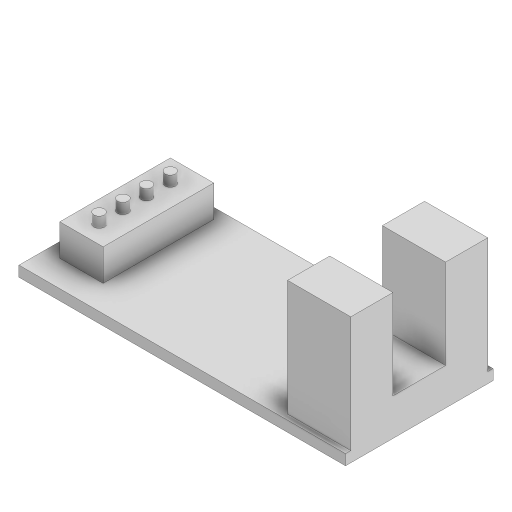
# Autodesk Inventor part: LM393
Saved by Autodesk Inventor 2024 (Build 280153000, 153)
## iProperties
Created: 2024-06-06
Part Number: LM393
Material: 一般
Document SubType Name: Modeling
Designer: USER
Density: 1 g/cm^3
Appearance: 預設
Author: USER
Autodesk Inventor part; units mm, degrees
ref_plane "YZ Plane" through (0, 0, 0) normal (1, 0, 0) x (0, 1, 0)
ref_plane "XZ Plane" through (0, 0, 0) normal (0, 1, 0) x (-1, 0, 0)
ref_plane "XY Plane" through (0, 0, 0) normal (0, 0, 1) x (1, 0, 0)
sketch "草圖1" plane through (0, 0, 0) normal (0, 1, 0) x (-1, 0, 0)
  line L0 (0, 0) -> (31, 0)
  line L1 (31, 0) -> (31, -14)
  line L2 (31, -14) -> (0, -14)
  line L3 (0, -14) -> (0, 0)
  line L4 (6, 0) -> (6, -14)
  line L5 (6, -0.5) -> (0, -0.5)
  line L6 (6, -4.5) -> (0, -4.5)
  line L7 (6, -13.5) -> (0, -13.5)
  line L8 (6, -9.5) -> (0, -9.5)
  line L9 (29.6283, -2.5) -> (25.5101, -2.5)
  line L10 (25.5101, -2.5) -> (25.5101, -13)
  line L11 (25.5101, -13) -> (29.6283, -13)
  line L12 (29.6283, -13) -> (29.6283, -2.5)
  dimension "d0" = 31
  dimension "d1" = 14
  dimension "d2" = 6
  dimension "d3" = 0.5
  dimension "d4" = 4
  dimension "d5" = 4
  dimension "d6" = 0.5
  dimension "d7" = 1
  dimension "d8" = 2.5
  constraints: 26 end point, 10 point on line, 5 parallel, 5 perpendicular, 2 horizontal, 1 vertical
  measures "d0" distance of L1.end L2.end
  measures "d1" distance of L2.end L0.start
  measures "d2" distance between parallel lines of L3 L4
  measures "d3" distance between parallel lines of L0 L5
  measures "d4" distance between parallel lines of L5 L6
  measures "d5" distance between parallel lines of L8 L7
  measures "d6" distance between parallel lines of L2 L7
  measures "d7" distance between parallel lines of L2 L11
  measures "d8" distance between parallel lines of L0 L9
extrude "擠出1" add sketch "草圖1" along normal blind 1 contours L0 L4 L5 L3 | L0 L1 L2 L4 | L5 L4 L6 L3 | L6 L4 L8 L3 | L8 L4 L7 L3 | L2 L3 L7 L4 | L12 L11 L10 L9
extrude "擠出2" add sketch "草圖1" along normal blind 12 contours L5 L4 L6 L3 | L8 L4 L7 L3
extrude "擠出3" add sketch "草圖1" along normal blind 4 contours L12 L11 L10 L9
sketch "草圖2" plane through (0, 4, 0) normal (0, 1, 0) x (1, 0, 0)
  circle A0 centre (-27.5692, 4.175) radius 0.5
  line L0 (-29.6283, 2.5) -> (-25.5101, 2.5) projected
  line L1 (-27.5692, 4.175) -> (-27.5692, 13)
  line L2 (-29.6283, 13) -> (-25.5101, 13) projected
  circle A1 centre (-27.5692, 6.425) radius 0.5
  circle A2 centre (-27.5692, 8.675) radius 0.5
  circle A3 centre (-27.5692, 10.925) radius 0.5
  point P0 (0, 0)
  point P1 (-27.5692, 2.5)
  dimension "d15" = 1
  dimension "d16" = 1.675
  dimension "d19" = 2.25
  constraints: 4 centre point, 2 end point, 2 midpoint, 1 vertical, 1 vertical alignment, 6 other
  measures "d15" diameter of A0
  measures "d16" distance from line of L0 L1.start
  measures "d19" distance of L1.start A1.centre
extrude "擠出4" add sketch "草圖2" along normal blind 1
extrude "擠出5" add sketch "草圖1" along normal blind 3.5 contours L6 L4 L8 L3
